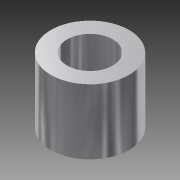
# Autodesk Inventor part: AS38-12-20
Saved by Autodesk Inventor 2014 (Build 180170000, 170)
## iProperties
Created: 2013-07-17
Part Number: AS38-12-20
Material: Aluminum 6061
Document SubType Name: Modeling
Designer: Edward
Density: 2.71 g/cm^3
Appearance: Aluminum - Polished
Catalog Web Link: 0.10
Vendor: Aluminum Spacer #AS38-12-20
Stock Number: AS38-12-20
d0: 5.560 mm
d1: 9.530 mm
d2: 7.940 mm
d3: 0.00 deg
Author: Edward
Autodesk Inventor part; units mm, degrees
ref_plane "YZ Plane" through (0, 0, 0) normal (1, 0, 0) x (0, 1, 0)
ref_plane "XZ Plane" through (0, 0, 0) normal (0, 1, 0) x (-1, 0, 0)
ref_plane "XY Plane" through (0, 0, 0) normal (0, 0, 1) x (1, 0, 0)
sketch "Sketch1" plane through (0, 0, 0) normal (0, 0, 1) x (1, 0, 0)
  circle A0 centre (0, 0) radius 2.78
  circle A1 centre (0, 0) radius 4.765
  dimension "d0" = 5.56
  dimension "d1" = 9.53
  constraints: 2 centre point, 2 coincident
  measures "d0" diameter of A0
  measures "d1" diameter of A1
extrude "Extrusion1" add sketch "Sketch1" along normal blind 7.94
body "Solid1"
